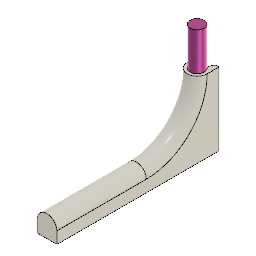
flex pitot cover v5 (Autodesk Fusion 360 design; units mm, degrees)
Autodesk Fusion 360 part; units mm, degrees
sketch "Sketch1" plane through (0, 0, 0) normal (0, 1, 0) x (1, 0, 0)
  circle A0 centre (7.25, -5.0145) radius 3.75
  circle A1 centre (7.25, -5.0145) radius 5.25
  line L0 (2, -5.0145) -> (12.5, -5.0145)
  line L1 (12.5, -5.0145) -> (12.5, 1.2355)
  line L2 (12.5, 1.2355) -> (2, 1.2355)
  line L3 (2, 1.2355) -> (2, -5.0145)
  dimension "d4" = 7.5
  dimension "d5" = 10.5
  dimension "d6" = 10.5
  dimension "d7" = 6.25
  constraint concentric A0 A1
  constraint horizontal L0
  constraint vertical L1
  constraint horizontal L2
  constraint vertical L3
  constraint coincident A1 L0.start
  constraint tangent A1 L3
  measures "d4" diameter of A0
  measures "d5" diameter of A1
  measures "d6" distance of L0.start L0.end
  measures "d7" distance of L0.start L2.end
extrude "Extrude1" add sketch "Sketch1" along normal blind 45 contours A0 A1 L0 | A0 A1 L0 | A1 L1 L2 L3 makes body 1
extrude "Extrude2" add sketch "Sketch1" against normal blind 2 bodies 1
sketch "Sketch2" plane through (0, 45, 0) normal (0, 1, 0) x (-1, 0, 0)
  circle A0 centre (-7.25, 5.0145) radius 3.75
  circle A1 centre (-7.25, 5.0145) radius 3.75
  line L0 (-7.25, 5.0145) -> (-7.25, 37.0145) construction
  line L1 (-25, 37.0145) -> (15, 37.0145) construction
  line L2 (-11, 5.0145) -> (-11, -1.2355)
  line L3 (-3.5, 5.0145) -> (-3.5, -1.2355)
  line L4 (-11, -1.2355) -> (-3.5, -1.2355)
  arc A2 (-2, 5.0145) -> (-12.5, 5.0145) centre (-7.25, 5.0145) ccw
  line L5 (-12.5, 5.0145) -> (-12.5, -1.2355)
  line L6 (-12.5, -1.2355) -> (-2, -1.2355)
  line L7 (-2, -1.2355) -> (-2, 5.0145)
  line L8 (-11, -1.2355) -> (-3.5, -1.2355)
  line L9 (-3.5, -1.2355) -> (-3.5, -45)
  line L10 (-3.5, -45) -> (-11, -45)
  line L11 (-11, -45) -> (-11, -1.2355)
  dimension "d12" = 7.5
  dimension "d13" = 32
  constraint concentric A0 A1
  constraint coincident A0.centre A1.centre
  constraint vertical L0
  constraint horizontal L1
  constraint coincident L0.end L1
  constraint coincident A1 L2.start
  constraint coincident A0 L3.start
  constraint tangent A1 L2
  constraint tangent A1 L3
  constraint coincident L2.end L6
  constraint coincident L3.end L6
  constraint vertical L2
  constraint horizontal L8
  constraint vertical L9
  constraint horizontal L10
  constraint vertical L11
  constraint coincident L3.end L9
  measures "d12" diameter of A1
  measures "d13" distance of A0.centre L0.end
revolve "Revolve2" add sketch "Sketch2" angle 90 about axis through (25, 45, 37.0145) along (1, 0, 0) contours A0 A1 L2 L3 L4 L6 L8 | A0 A1 L2 L3 A2 L5 L6 L7 bodies 1
sketch "Sketch8" plane through (2, 0, 0) normal (-1, 0, 0) x (0, -1, 0)
  line L0 (2, 5.0145) -> (-45, 5.0145)
  arc A0 (-77, 37.0145) -> (-45, 5.0145) centre (-45, 37.0145) ccw
  line L1 (-77, 37.0145) -> (-83.25, 37.0145)
  arc A1 (-83.25, 37.0145) -> (-45, -1.2355) centre (-45, 37.0145) ccw
  line L2 (-45, -1.2355) -> (2, -1.2355)
  line L3 (2, -1.2355) -> (2, 5.0145)
  line L4 (-45, -1.2355) -> (-83.25, -1.2355)
  line L5 (-83.25, -1.2355) -> (-83.25, 37.0145)
  line L6 (-83.25, 37.0145) -> (-45, 37.0145)
  line L7 (-45, 37.0145) -> (-45, -1.2355)
  constraint horizontal L4
  constraint vertical L5
  constraint horizontal L6
  constraint vertical L7
  constraint coincident L1.end A1.start
  constraint coincident A1.end L2.start
extrude "Extrude8" add sketch "Sketch8" against normal up to surface (10.5 mm away) contours A1 L4 L5 bodies 1
revolve "Revolve3" cut sketch "Sketch2" angle 90 about axis through (25, 45, 37.0145) along (1, 0, 0) contours A0 A1 | A0 A1 L2 L3 L4 L6 L8 | L4 L6 L8 L9 L10 L11 bodies 1
sketch "Sketch3" plane through (0, 0, 37.0145) normal (0, 0, 1) x (-1, 0, 0)
  line L0 (-3.5, -77) -> (-3.5, -83.25)
  line L1 (-11, -83.25) -> (-11, -77)
  arc A0 (-3.5, -77) -> (-11, -77) centre (-7.25, -77) ccw
  line L2 (-3.5, -79.7034) -> (-2, -79.7034)
  line L3 (-2, -79.7034) -> (-2, -83.25)
  line L4 (-2, -83.25) -> (-3.5, -83.25)
  line L5 (-3.5, -83.25) -> (-3.5, -79.7034)
  line L6 (-2, -83.25) -> (-2, -77)
  arc A1 (-2, -77) -> (-12.5, -77) centre (-7.25, -77) ccw
  line L7 (-12.5, -77) -> (-12.5, -83.25)
  line L8 (-3.5, -83.25) -> (-2, -83.25)
  line L9 (-12.5, -83.25) -> (-11, -83.25)
  constraint horizontal L2
  constraint vertical L3
  constraint horizontal L4
  constraint vertical L5
  constraint coincident L0.end L4.end
sketch "Sketch4" plane through (3.5, 0, 0) normal (1, 0, 0) x (0, 1, 0)
  line L0 (45, 5.0145) -> (45, -1.2355)
  arc A0 (45, 5.0145) -> (77, 37.0145) centre (45, 37.0145) ccw
  line L1 (81.0767, 47.3152) -> (81.8767, 47.3152)
  line L2 (81.8767, 47.3152) -> (81.8767, 45.3152)
  line L3 (81.8767, 45.3152) -> (81.0767, 45.3152)
  line L4 (81.0767, 45.3152) -> (81.0767, 47.3152)
  line L5 (81.0767, 46.3152) -> (79.7034, 46.3152) construction
  line L6 (81.8767, 46.3152) -> (83.25, 46.3152) construction
  line L7 (83.25, 37.0145) -> (77, 37.0145)
  line L8 (45, -1.2355) -> (83.25, -1.2355)
  line L9 (83.25, -1.2355) -> (83.25, 37.0145)
  dimension "d28" = 0.8
  dimension "d29" = 2
  constraint horizontal L1
  constraint vertical L2
  constraint horizontal L3
  constraint vertical L4
  constraint midpoint L4 L5.start
  constraint midpoint L2 L6.start
  constraint equal L5 L6
  measures "d28" distance of L1.start L1.end
  measures "d29" distance of L1.start L3.end
extrude "Extrude4" add sketch "Sketch1" along normal blind 45 separate body contours A0 L0 | A0 L0 makes body 2
revolve "Revolve4" add sketch "Sketch2" angle 90 about axis through (25, 45, 37.0145) along (1, 0, 0) contours A0 A1 bodies 2
extrude "Extrude5" add 1 faces at (8.3762, 76.4576, 37.0145) along direction (0, 0, 1) blind 20 on bodies 2 bodies 2
ref_plane "WorkPlane1" through (7.25, 40.625, 17.8895) normal (1, 0, 0) x (0, 0, -1)
sketch "Sketch9" plane through (0, 0, -1.2355) normal (0, 0, -1) x (1, 0, 0)
  line L0 (3.5, -83.25) -> (3.5, -45)
  line L1 (3.5, -45) -> (11, -45)
  line L2 (11, -45) -> (11, -83.25)
  line L3 (11, -83.25) -> (12.5, -83.25)
  line L4 (12.5, -83.25) -> (12.5, 2)
  line L5 (12.5, 2) -> (2, 2)
  line L6 (2, 2) -> (2, -83.25)
  line L7 (2, -83.25) -> (3.5, -83.25)
  arc A0 (3.5, -83.25) -> (3.5, -77.25) centre (1.2708, -80.25) ccw
  dimension "d45" = 6
  constraint coincident L0 A0.end
  constraint coincident L0.start L7.end
  measures "d45" distance of L0.start A0.end
extrude "Extrude9" add sketch "Sketch9" against normal up to surface (38.25 mm away) contours L0 A0 bodies 1
mirror "Mirror1" about plane through (7.25, 40.625, 17.8895) normal (1, 0, 0) of "Extrude9"
equation "pitotdiameter = 7.5 mm"
equation "pitotlength = 45 mm"
equation "bendid = 32 mm"
equation "d4 = pitotdiameter"
equation "d5 = pitotdiameter + 3 mm"
equation "d6 = pitotdiameter + 3 mm"
equation "d7 = ( pitotdiameter / 2 ) + 2.5 mm"
equation "d8 = pitotlength"
equation "d12 = pitotdiameter"
equation "d13 = bendid"
equation "d21 = pitotlength"
equation "shellthickness = 4 mm"
named bodies: "cover", "pitot"
